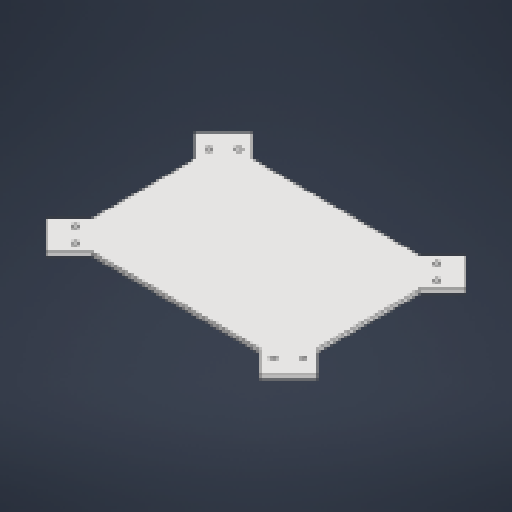
# Autodesk Inventor part: electronics panel
Saved by Autodesk Inventor 2023 (Build 270158000, 158)
## iProperties
Created: 2023-01-16
Part Number: electronics panel
Material: Generic
Document SubType Name: Modeling
Designer: Michael
Density: 1 g/cm^3
Appearance: Default
Author: Michael
Autodesk Inventor part; units mm, degrees
ref_plane "YZ Plane" through (0, 0, 0) normal (1, 0, 0) x (0, 1, 0)
ref_plane "XZ Plane" through (0, 0, 0) normal (0, 1, 0) x (-1, 0, 0)
ref_plane "XY Plane" through (0, 0, 0) normal (0, 0, 1) x (1, 0, 0)
sketch "Sketch2" plane through (0, 0, 0) normal (0, 1, 0) x (-1, 0, 0)
  line L0 (0, 0) -> (177.8, 0)
  line L1 (177.8, 0) -> (177.8, -127)
  line L2 (177.8, -127) -> (0, -127)
  line L3 (0, -127) -> (0, 0)
  line L4 (155.3506, 0) -> (177.8, -22.4519) projected
  line L5 (177.8, -104.5481) -> (155.3506, -127) projected
  line L6 (0, -22.4519) -> (22.4494, 0) projected
  line L7 (22.4494, -127) -> (0, -104.5481) projected
  line L8 (155.3506, 0) -> (173.3121, 17.9595)
  line L9 (173.3121, 17.9595) -> (195.7615, -4.4923)
  line L10 (195.7615, -4.4923) -> (177.8, -22.4519)
  line L11 (177.8, -63.5) -> (0, -63.5)
  line L12 (88.9, -127) -> (88.9, 0)
  line L13 (155.3506, -127) -> (177.8, -104.5481)
  line L14 (155.3506, -127) -> (173.3121, -144.9595)
  line L15 (173.3121, -144.9595) -> (195.7615, -122.5077)
  line L16 (195.7615, -122.5077) -> (177.8, -104.5481)
  line L17 (22.4494, 0) -> (0, -22.4519)
  line L18 (0, -104.5481) -> (22.4494, -127)
  line L19 (22.4494, 0) -> (4.4879, 17.9595)
  line L20 (4.4879, 17.9595) -> (-17.9615, -4.4923)
  line L21 (-17.9615, -4.4923) -> (0, -22.4519)
  line L22 (4.4879, -144.9595) -> (-17.9615, -122.5077)
  line L23 (22.4494, -127) -> (4.4879, -144.9595)
  line L24 (-17.9615, -122.5077) -> (0, -104.5481)
  circle A0 centre (178.6987, -10.7776) radius 2.2479 projected
  circle A1 centre (167.025, 0.8974) radius 2.2479 projected
  circle A2 centre (178.6987, -116.2224) radius 2.2479 projected
  circle A3 centre (167.025, -127.8974) radius 2.2479 projected
  circle A4 centre (10.775, 0.8974) radius 2.2479 projected
  circle A5 centre (-0.8987, -10.7776) radius 2.2479 projected
  circle A6 centre (-0.8987, -116.2224) radius 2.2479 projected
  circle A7 centre (10.775, -127.8974) radius 2.2479 projected
  dimension "d0" = 177.8
  dimension "d1" = 127
  dimension "d30" = 25.4
  constraints: 42 end point, 6 symmetric about line, 4 midpoint, 3 perpendicular, 2 parallel, 1 horizontal
  measures "d0" distance of L1.end L2.end
  measures "d1" distance of L0.end L1.end
  measures "d30" distance of L4.start L8.end
extrude "Extrusion8" add sketch "Sketch2" against normal blind 3.175 contours L6 L3 A5 L0 A4 | L0 L12 L11 L3 L6 | L0 A4 L3 A5 L21 L20 L19 | L0 L4 L1 L11 L12 | L8 L9 L10 L1 A0 L0 A1 | L0 A1 L1 A0 L4 | L12 L2 L7 L3 L11 | L11 L1 L5 L2 L12 | L7 L2 A7 L3 A6 | L3 A6 L2 A7 L23 L22 L24 | L16 L15 L14 L2 A3 L1 A2 | L1 A2 L2 A3 L5
body "Solid3"
